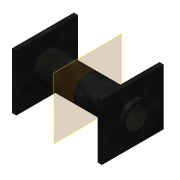
# Autodesk Inventor part: frame
Saved by Autodesk Inventor 2018.1 (Build 221171000, 171)
## iProperties
Created: 2019-06-27
Part Number: frame
Material: Пластмасса, непрозрачная, черная
Document SubType Name: Modeling
Designer: Boss
Mass: 1.94751 g
Surface Area: 35.828 cm^2
Volume: 2.04571 cm^3
Density: 0.952 g/cm^3
Appearance: Гладкая — черная
Author: Boss
Autodesk Inventor part; units mm, degrees
ref_plane "YZ Plane" through (0, 0, 0) normal (1, 0, 0) x (0, 1, 0)
ref_plane "XZ Plane" through (0, 0, 0) normal (0, 1, 0) x (-1, 0, 0)
ref_plane "XY Plane" through (0, 0, 0) normal (0, 0, 1) x (1, 0, 0)
sketch "Эскиз1" plane through (0, 0, 0) normal (1, 0, 0) x (0, 1, 0)
  line L0 (-11, 10) -> (11, 10)
  line L1 (11, 10) -> (11, -10)
  line L2 (11, -10) -> (-11, -10)
  line L3 (-11, -10) -> (-11, 10)
  line L4 (-11, 10) -> (11, -10) construction
  line L5 (11, 10) -> (-11, -10) construction
  circle A0 centre (0, 0) radius 5
  dimension "d1" = 22
  dimension "d2" = 20
  dimension "d3" = 10
  constraints: 12 end point, 2 midpoint, 2 parallel, 1 centre point, 1 coincident, 1 horizontal, 1 perpendicular
  measures "d1" distance of L1.end L2.end
  measures "d2" distance of L0.end L1.end
  measures "d3" diameter of A0
extrude "Выдавливание1" add sketch "Эскиз1" along normal blind 1.5
ref_plane "РабПлоскость1" through (16, 0, 0) normal (1, 0, 0) x (0, 0, -1)
mirror "Зеркальное отражение1" about plane through (16, 0, 0) normal (1, 0, 0) of "Выдавливание1"
sketch "Эскиз2" plane through (0, 0, 0) normal (-1, 0, 0) x (0, 0, 1)
  circle A0 centre (0, 0) radius 5 projected
  circle A1 centre (0, 0) radius 4
  dimension "d7" = 8
  constraints: 1 centre point, 1 coincident
  measures "d7" diameter of A1
extrude "Выдавливание2" add sketch "Эскиз2" against normal blind 34
